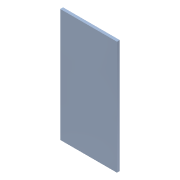
# Autodesk Inventor part: coverSlip_5mmX10mm
Saved by Autodesk Inventor 2014 (Build 180170000, 170)
## iProperties
Created: 2016-08-15
Part Number: coverSlip_5mmX10mm
Material: Generic
Document SubType Name: Modeling
Designer: Camilo
Density: 1 g/cm^3
Appearance: Blue - Glazing
Author: Camilo
Autodesk Inventor part; units mm, degrees
ref_plane "YZ Plane" through (0, 0, 0) normal (1, 0, 0) x (0, 1, 0)
ref_plane "XZ Plane" through (0, 0, 0) normal (0, 1, 0) x (-1, 0, 0)
ref_plane "XY Plane" through (0, 0, 0) normal (0, 0, 1) x (1, 0, 0)
sketch "Sketch1" plane through (0, 0, 0) normal (0, 1, 0) x (-1, 0, 0)
  line L0 (-2.5, -5) -> (2.5, -5)
  line L1 (2.5, -5) -> (2.5, 5)
  line L2 (2.5, 5) -> (-2.5, 5)
  line L3 (-2.5, 5) -> (-2.5, -5)
  line L4 (-2.5, -5) -> (2.5, 5) construction
  line L5 (2.5, -5) -> (-2.5, 5) construction
  point P0 (0, 0)
  constraints: 12 end point, 2 midpoint
extrude "Extrusion1" add sketch "Sketch1" along normal blind 0.25
body "Solid1"
